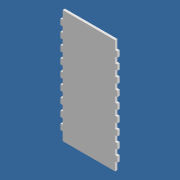
# Autodesk Inventor part: BackFrontPannel
Saved by Autodesk Inventor 2021 (Build 250183000, 183)
## iProperties
Created: 2022-09-19
Part Number: BackFrontPannel
Material: Generic
Document SubType Name: Modeling
Designer: Nathann
Density: 1 g/cm^3
Appearance: Default
Author: Nathann
Autodesk Inventor part; units mm, degrees
ref_plane "YZ Plane" through (0, 0, 0) normal (1, 0, 0) x (0, 1, 0)
ref_plane "XZ Plane" through (0, 0, 0) normal (0, 1, 0) x (-1, 0, 0)
ref_plane "XY Plane" through (0, 0, 0) normal (0, 0, 1) x (1, 0, 0)
sketch "Sketch1" plane through (0, 0, 0) normal (0, 0, 1) x (1, 0, 0)
  line L0 (0, 0) -> (162, 0)
  line L1 (162, 0) -> (162, -300)
  line L2 (162, -300) -> (0, -300)
  line L3 (0, -300) -> (0, 0)
  dimension "d0" = 162
  dimension "d1" = 300
  constraints: 8 end point, 2 parallel, 1 horizontal, 1 perpendicular
  measures "d0" distance of L0.start L0.end
  measures "d1" distance of L2.end L0.start
extrude "Extrusion1" add sketch "Sketch1" along normal blind 6
sketch "Sketch2" plane through (0, 0, 0) normal (0, 0, -1) x (-1, 0, 0)
  line L0 (0, 0) -> (-5.9, 0)
  line L1 (-5.9, 0) -> (-5.9, -22.5)
  line L2 (-5.9, -22.5) -> (0, -22.5)
  line L3 (0, -22.5) -> (0, 0)
  line L4 (-162, 0) -> (0, 0) projected
  line L5 (0, 0) -> (0, -300) projected
  line L6 (0, -37.5) -> (-5.9, -37.5)
  line L7 (-5.9, -37.5) -> (-5.9, -52.5)
  line L8 (-5.9, -52.5) -> (0, -52.5)
  line L9 (0, -52.5) -> (0, -37.5)
  line L10 (0, -30) -> (-5.9, -30)
  line L11 (0, -67.5) -> (-5.9, -67.5)
  line L12 (-5.9, -67.5) -> (-5.9, -82.5)
  line L13 (-5.9, -82.5) -> (0, -82.5)
  line L14 (0, -82.5) -> (0, -67.5)
  line L15 (0, -60) -> (-5.9, -60)
  line L16 (0, -97.5) -> (-5.9, -97.5)
  line L17 (-5.9, -97.5) -> (-5.9, -112.5)
  line L18 (-5.9, -112.5) -> (0, -112.5)
  line L19 (0, -112.5) -> (0, -97.5)
  line L20 (0, -90) -> (-5.9, -90)
  line L21 (0, -127.5) -> (-5.9, -127.5)
  line L22 (-5.9, -127.5) -> (-5.9, -142.5)
  line L23 (-5.9, -142.5) -> (0, -142.5)
  line L24 (0, -142.5) -> (0, -127.5)
  line L25 (0, -120) -> (-5.9, -120)
  line L26 (0, -157.5) -> (-5.9, -157.5)
  line L27 (-5.9, -157.5) -> (-5.9, -172.5)
  line L28 (-5.9, -172.5) -> (0, -172.5)
  line L29 (0, -172.5) -> (0, -157.5)
  line L30 (0, -150) -> (-5.9, -150)
  line L31 (0, -187.5) -> (-5.9, -187.5)
  line L32 (-5.9, -187.5) -> (-5.9, -202.5)
  line L33 (-5.9, -202.5) -> (0, -202.5)
  line L34 (0, -202.5) -> (0, -187.5)
  line L35 (0, -180) -> (-5.9, -180)
  line L36 (0, -217.5) -> (-5.9, -217.5)
  line L37 (-5.9, -217.5) -> (-5.9, -232.5)
  line L38 (-5.9, -232.5) -> (0, -232.5)
  line L39 (0, -232.5) -> (0, -217.5)
  line L40 (0, -210) -> (-5.9, -210)
  line L41 (0, -247.5) -> (-5.9, -247.5)
  line L42 (-5.9, -247.5) -> (-5.9, -262.5)
  line L43 (-5.9, -262.5) -> (0, -262.5)
  line L44 (0, -262.5) -> (0, -247.5)
  line L45 (0, -300) -> (-5.9, -300)
  line L46 (-5.9, -300) -> (-5.9, -277.5)
  line L47 (-5.9, -277.5) -> (0, -277.5)
  line L48 (0, -277.5) -> (0, -300)
  line L49 (-162, 0) -> (0, 0) projected
  line L50 (-81, 0) -> (-81, -60)
  line L51 (-162, 0) -> (-156.1, 0)
  line L52 (-156.1, 0) -> (-156.1, -22.5)
  line L53 (-156.1, -22.5) -> (-162, -22.5)
  line L54 (-162, -22.5) -> (-162, 0)
  line L55 (0, 0) -> (-162, 0)
  line L56 (-162, 0) -> (-162, -300)
  line L57 (-162, -37.5) -> (-156.1, -37.5)
  line L58 (-156.1, -37.5) -> (-156.1, -52.5)
  line L59 (-156.1, -52.5) -> (-162, -52.5)
  line L60 (-162, -52.5) -> (-162, -37.5)
  line L61 (-162, -30) -> (-156.1, -30)
  line L62 (-162, -67.5) -> (-156.1, -67.5)
  line L63 (-156.1, -67.5) -> (-156.1, -82.5)
  line L64 (-156.1, -82.5) -> (-162, -82.5)
  line L65 (-162, -82.5) -> (-162, -67.5)
  line L66 (-162, -60) -> (-156.1, -60)
  line L67 (-162, -97.5) -> (-156.1, -97.5)
  line L68 (-156.1, -97.5) -> (-156.1, -112.5)
  line L69 (-156.1, -112.5) -> (-162, -112.5)
  line L70 (-162, -112.5) -> (-162, -97.5)
  line L71 (-162, -90) -> (-156.1, -90)
  line L72 (-162, -127.5) -> (-156.1, -127.5)
  line L73 (-156.1, -127.5) -> (-156.1, -142.5)
  line L74 (-156.1, -142.5) -> (-162, -142.5)
  line L75 (-162, -142.5) -> (-162, -127.5)
  line L76 (-162, -120) -> (-156.1, -120)
  line L77 (-162, -157.5) -> (-156.1, -157.5)
  line L78 (-156.1, -157.5) -> (-156.1, -172.5)
  line L79 (-156.1, -172.5) -> (-162, -172.5)
  line L80 (-162, -172.5) -> (-162, -157.5)
  line L81 (-162, -150) -> (-156.1, -150)
  line L82 (-162, -187.5) -> (-156.1, -187.5)
  line L83 (-156.1, -187.5) -> (-156.1, -202.5)
  line L84 (-156.1, -202.5) -> (-162, -202.5)
  line L85 (-162, -202.5) -> (-162, -187.5)
  line L86 (-162, -180) -> (-156.1, -180)
  line L87 (-162, -217.5) -> (-156.1, -217.5)
  line L88 (-156.1, -217.5) -> (-156.1, -232.5)
  line L89 (-156.1, -232.5) -> (-162, -232.5)
  line L90 (-162, -232.5) -> (-162, -217.5)
  line L91 (-162, -210) -> (-156.1, -210)
  line L92 (-162, -247.5) -> (-156.1, -247.5)
  line L93 (-156.1, -247.5) -> (-156.1, -262.5)
  line L94 (-156.1, -262.5) -> (-162, -262.5)
  line L95 (-162, -262.5) -> (-162, -247.5)
  line L96 (-162, -300) -> (-156.1, -300)
  line L97 (-156.1, -300) -> (-156.1, -277.5)
  line L98 (-156.1, -277.5) -> (-162, -277.5)
  line L99 (-162, -277.5) -> (-162, -300)
  line L100 (0, 0) -> (-162, 0)
  point P0 (-162, -277.5)
  point P1 (0, -277.5)
  point P2 (0, -262.5)
  point P3 (0, -232.5)
  point P4 (0, -202.5)
  point P5 (-162, -82.5)
  point P6 (0, -172.5)
  point P7 (-162, -157.5)
  point P8 (0, -142.5)
  point P9 (-162, -142.5)
  point P10 (0, -112.5)
  point P11 (-162, -97.5)
  point P12 (0, -82.5)
  point P13 (-162, -247.5)
  point P14 (-156.1, 0)
  point P15 (-162, -232.5)
  dimension "d4" = 0
  dimension "d5" = 5.9
  dimension "d6" = 0
  dimension "d7" = 22.5
  dimension "d8" = 5.9
  dimension "d9" = 15
  dimension "d10" = 15
  dimension "d13" = 30
  dimension "d18" = 22.5
  dimension "d19" = 5.9
  constraints: 196 end point, 56 symmetric about line, 6 parallel, 3 horizontal, 3 perpendicular, 2 point on line, 2 vertical, 1 midpoint, 77 other
  measures "d4" distance between parallel lines of L4 L0
  measures "d5" distance of L1.end L2.end
  measures "d6" distance between parallel lines of L5 L3
  measures "d7" distance of L0.end L1.end
  measures "d8" distance of L6.start L6.end
  measures "d9" distance of L6.end L7.end
  measures "d10" distance between parallel lines of L6 L2
  measures "d13" distance of L0.start L10.start
  measures "d18" distance of L45.end L46.end
  measures "d19" distance of L46.end L47.end
extrude "Extrusion2" cut sketch "Sketch2" against normal mid plane 24
sketch "Sketch3" plane through (0, 0, 6) normal (0, 0, 1) x (1, 0, 0)
  circle A0 centre (28.4, -30) radius 2.5
  circle A1 centre (133.4, -30) radius 2.5
  circle A2 centre (28.4, -135) radius 2.5
  circle A3 centre (133.4, -135) radius 2.5
  circle A4 centre (28.4, -165) radius 2.5
  circle A5 centre (133.4, -165) radius 2.5
  circle A6 centre (28.4, -270) radius 2.5
  circle A7 centre (133.4, -270) radius 2.5
  line L0 (5.9, 0) -> (5.9, -22.5) projected
  line L1 (156.1, -22.5) -> (156.1, 0) projected
  line L2 (5.9, -300) -> (156.1, -300) projected
  line L3 (156.1, 0) -> (5.9, 0) projected
  circle A8 centre (81, -82.5) radius 56.9012
  circle A9 centre (81, -217.5) radius 58.271
  line L4 (156.1, -202.5) -> (156.1, -187.5) projected
  point P0 (0, 0)
  dimension "d22" = 5
  dimension "d23" = 5
  dimension "d24" = 5
  dimension "d25" = 5
  dimension "d26" = 5
  dimension "d27" = 5
  dimension "d28" = 5
  dimension "d29" = 5
  dimension "d30" = 105
  dimension "d31" = 105
  dimension "d32" = 105
  dimension "d33" = 22.5
  dimension "d34" = 150.2
  dimension "d35" = 105
  dimension "d36" = 105
  dimension "d37" = 105
  dimension "d38" = 30
  dimension "d39" = 22.5
  dimension "d40" = 30
  dimension "d41" = 105
  dimension "d44" = 135
  dimension "d45" = 30
  dimension "d46" = 82.5
  dimension "d47" = 75.1
  dimension "d48" = 75.1
  constraints: 10 centre point, 3 vertical alignment, 2 horizontal alignment
  measures "d22" diameter of A0
  measures "d23" diameter of A1
  measures "d24" diameter of A2
  measures "d25" diameter of A3
  measures "d26" diameter of A4
  measures "d27" diameter of A5
  measures "d28" diameter of A6
  measures "d29" diameter of A7
  measures "d30" distance of A1.centre A0.centre
  measures "d31" distance of A3.centre A2.centre
  measures "d32" distance of A2.centre A0.centre
  measures "d33" distance from line of L0 A0.centre
  measures "d34" distance between parallel lines of L1 L0
  measures "d35" distance of A5.centre A4.centre
  measures "d36" distance of A7.centre A6.centre
  measures "d37" distance of A6.centre A4.centre
  measures "d38" distance from line of L2 A6.centre
  measures "d39" distance from line of L0 A4.centre
  measures "d40" distance from line of L3 A0.centre
  measures "d41" distance of A7.centre A5.centre
  measures "d44" distance of A9.centre A8.centre
  measures "d45" distance of A5.centre A3.centre
  measures "d46" distance from line of L3 A8.centre
  measures "d47" distance from line of L4 A9.centre
  measures "d48" distance from line of L0 A8.centre
extrude "Extrusion3" cut sketch "Sketch3" along normal mid plane 24
equation "\"d2\" = WoodWidth"
equation "\"d5\" = WoodWidth - LaserWith"
equation "\"d8\" = d5"
equation "\"d18\" = d7"
equation "\"d19\" = d5"
equation "\"d20\" = 4 * WoodWidth"
equation "\"d39\" = d33"
equation "\"d40\" = d38"
equation "\"d42\" = 4 * WoodWidth"
equation "\"WoodWidth\" = 6"
equation "\"LaserWith\" = 0.1"
body "Solid1"
